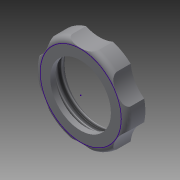
# Autodesk Inventor part: Крышка
Saved by Autodesk Inventor 2014 SP1 (Build 180222100, 222)
## iProperties
Created: 2023-07-18
Part Number: Крышка
Material: Типовые
Document SubType Name: Modeling
Designer: 1.507-7
Density: 1 g/cm^3
Appearance: По умолчанию
Author: 1.507-7
Autodesk Inventor part; units mm, degrees
ref_plane "YZ Plane" through (0, 0, 0) normal (1, 0, 0) x (0, 1, 0)
ref_plane "XZ Plane" through (0, 0, 0) normal (0, 1, 0) x (-1, 0, 0)
ref_plane "XY Plane" through (0, 0, 0) normal (0, 0, 1) x (1, 0, 0)
sketch "Эскиз1" plane through (0, 0, 0) normal (1, 0, 0) x (0, 1, 0)
  line L0 (0, 0) -> (0, 30)
  line L1 (0, 0) -> (4, 0)
  line L2 (4, 0) -> (4, 26)
  line L3 (4, 26) -> (14, 26)
  line L4 (14, 26) -> (14, 34)
  line L5 (14, 34) -> (4, 34)
  arc A0 (4, 34) -> (0, 30) centre (4, 30) ccw
  point P0 (0, 30)
  dimension "d2" = 4
  constraints: 12 end point, 4 perpendicular, 2 point on circle, 2 point on line, 2 tangent, 1 centre point, 1 parallel, 1 vertical
  measures "d2" distance of L0.start L1.end
revolve "Вращение1" add sketch "Эскиз1" angle 360 about axis through (0, 0, 0) along (0, 1, 0)
sketch "Эскиз2" plane through (0, 0, 0) normal (0, -1, 0) x (1, 0, 0)
  circle A0 centre (0, 0) radius 30 projected
sketch "Эскиз3" plane through (0, 0, 0) normal (0, -1, 0) x (1, 0, 0)
  circle A0 centre (0, 0) radius 30 projected
  circle A1 centre (0, 0) radius 30
  constraints: 1 centre point, 1 coincident, 1 concentric
hole "Отверстие1" at (0, 0, 0) direction (0, 1, 0) diameter 45 end through all
sketch "Эскиз4" plane through (0, 0, 0) normal (0, -1, 0) x (1, 0, 0)
  circle A0 centre (0, 0) radius 30 projected
  circle A1 centre (0, 55.1977) radius 24.8245
  circle A2 centre (47.8026, 27.5988) radius 24.8245
  circle A3 centre (47.8026, -27.5988) radius 24.8245
  circle A4 centre (0, -55.1977) radius 24.8245
  circle A5 centre (-47.8026, -27.5988) radius 24.8245
  circle A6 centre (-47.8026, 27.5988) radius 24.8245
  dimension "d18" = 360
  constraints: 6 centre point, 13 other
extrude "Выдавливание1" cut sketch "Эскиз4" along normal through all both and the other way through all contours A1 | A2 | A3 | A4 | A5 | A6
thread "Резьба1" size "M52x5" class "6H" standard "ISO Metric profile" full length
